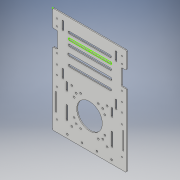
# Autodesk Inventor part: m600frontplate
Saved by Autodesk Inventor 2019 (Build 230136000, 136)
## iProperties
Created: 2019-07-15
Part Number: m600frontplate
Material: Generic
Document SubType Name: Modeling
Designer: Dell
Density: 1 g/cm^3
Appearance: Default
Author: Dell
Autodesk Inventor part; units mm, degrees
ref_plane "YZ Plane" through (0, 0, 0) normal (1, 0, 0) x (0, 1, 0)
ref_plane "XZ Plane" through (0, 0, 0) normal (0, 1, 0) x (-1, 0, 0)
ref_plane "XY Plane" through (0, 0, 0) normal (0, 0, 1) x (1, 0, 0)
sketch "Sketch1" plane through (0, 0, 0) normal (0, 0, 1) x (1, 0, 0)
  line L0 (0, 0) -> (150, 0)
  line L1 (150, 0) -> (150, -215)
  line L2 (150, -215) -> (0, -215)
  line L3 (0, -215) -> (0, 0)
  dimension "d0" = 150
  dimension "d1" = 215
  constraints: 8 end point, 2 parallel, 1 horizontal, 1 perpendicular
  measures "d0" distance of L1.end L2.end
  measures "d1" distance of L0.end L1.end
extrude "Extrusion1" add sketch "Sketch1" along normal blind 2
sketch "Sketch2" plane through (0, 0, 2) normal (0, 0, 1) x (1, 0, 0)
  line L0 (150, 0) -> (0, 0) projected
  line L1 (150, 0) -> (141.16, 0)
  line L2 (141.16, 0) -> (141.16, -27.95)
  line L3 (141.16, -27.95) -> (150, -27.95)
  line L4 (150, -27.95) -> (150, 0)
  line L5 (0, 0) -> (8.84, 0)
  line L6 (8.84, 0) -> (8.84, -27.95)
  line L7 (8.84, -27.95) -> (0, -27.95)
  line L8 (0, -27.95) -> (0, 0)
  line L9 (0, 0) -> (8.84, 0)
  line L10 (8.84, 0) -> (8.84, -13.975)
  line L11 (8.84, -13.975) -> (0, -13.975)
  line L12 (0, -13.975) -> (0, 0)
  line L13 (150, 0) -> (141.16, 0)
  line L14 (141.16, 0) -> (141.16, -13.975)
  line L15 (141.16, -13.975) -> (150, -13.975)
  line L16 (150, -13.975) -> (150, 0)
  circle A0 centre (141.16, -13.975) radius 1.3
  circle A1 centre (141.16, -27.95) radius 1.3
  circle A2 centre (8.84, -13.975) radius 1.3
  circle A3 centre (8.84, -27.95) radius 1.3
  line L17 (0, 0) -> (8.84, 0)
  line L18 (8.84, 0) -> (8.84, -75.2318)
  line L19 (8.84, -75.2318) -> (0, -75.2318)
  line L20 (0, -75.2318) -> (0, 0)
  line L21 (0, 0) -> (0, -215) projected
  line L22 (0, 0) -> (8.84, 0)
  line L23 (8.84, 0) -> (8.84, -95.1591)
  line L24 (8.84, -95.1591) -> (0, -95.1591)
  line L25 (0, -95.1591) -> (0, 0)
  line L26 (0, 0) -> (8.84, 0)
  line L27 (8.84, 0) -> (8.84, -113.5536)
  line L28 (8.84, -113.5536) -> (0, -113.5536)
  line L29 (0, -113.5536) -> (0, 0)
  line L30 (0, 0) -> (8.84, 0)
  line L31 (8.84, 0) -> (8.84, -134.4006)
  line L32 (8.84, -134.4006) -> (0, -134.4006)
  line L33 (0, -134.4006) -> (0, 0)
  line L34 (0, 0) -> (8.84, 0)
  line L35 (8.84, 0) -> (8.84, -192)
  line L36 (8.84, -192) -> (0, -192)
  line L37 (0, -192) -> (0, 0)
  line L38 (150, 0) -> (141.16, 0)
  line L39 (141.16, 0) -> (141.16, -75.2318)
  line L40 (141.16, -75.2318) -> (150, -75.2318)
  line L41 (150, -75.2318) -> (150, 0)
  line L42 (150, 0) -> (141.16, 0)
  line L43 (141.16, 0) -> (141.16, -95.1591)
  line L44 (141.16, -95.1591) -> (150, -95.1591)
  line L45 (150, -95.1591) -> (150, 0)
  line L46 (150, -215) -> (150, 0) projected
  line L47 (150, 0) -> (141.16, 0)
  line L48 (141.16, 0) -> (141.16, -113.5536)
  line L49 (141.16, -113.5536) -> (150, -113.5536)
  line L50 (150, -113.5536) -> (150, 0)
  line L51 (150, 0) -> (141.16, 0)
  line L52 (141.16, 0) -> (141.16, -134.4006)
  line L53 (141.16, -134.4006) -> (150, -134.4006)
  line L54 (150, -134.4006) -> (150, 0)
  line L55 (150, 0) -> (141.16, 0)
  line L56 (141.16, 0) -> (141.16, -192)
  line L57 (141.16, -192) -> (150, -192)
  line L58 (150, -192) -> (150, 0)
  circle A4 centre (8.84, -75.2318) radius 1.3
  circle A5 centre (141.16, -75.2318) radius 1.3
  circle A6 centre (141.16, -95.1591) radius 1.3
  circle A7 centre (8.84, -95.1591) radius 1.3
  circle A8 centre (8.84, -113.5536) radius 1.3
  circle A9 centre (141.16, -113.5536) radius 1.3
  circle A10 centre (141.16, -134.4006) radius 1.3
  circle A11 centre (8.84, -134.4006) radius 1.3
  circle A12 centre (141.16, -192) radius 1.3
  circle A13 centre (8.84, -192) radius 1.3
  line L59 (0, -27.95) -> (10.14, -27.95)
  line L60 (10.14, -27.95) -> (10.14, -34.95)
  line L61 (10.14, -34.95) -> (0, -34.95)
  line L62 (0, -34.95) -> (0, -27.95)
  line L63 (0, -75.2318) -> (10.14, -75.2318)
  line L64 (10.14, -75.2318) -> (10.14, -67.9551)
  line L65 (10.14, -67.9551) -> (0, -67.9551)
  line L66 (0, -67.9551) -> (0, -75.2318)
  line L67 (10.14, -34.95) -> (0, -34.95)
  line L68 (0, -34.95) -> (0, -67.9551)
  line L69 (0, -67.9551) -> (10.14, -67.9551)
  line L70 (10.14, -67.9551) -> (10.14, -34.95)
  line L71 (150, -27.95) -> (139.86, -27.95)
  line L72 (139.86, -27.95) -> (139.86, -34.95)
  line L73 (139.86, -34.95) -> (150, -34.95)
  line L74 (150, -34.95) -> (150, -27.95)
  line L75 (139.86, -34.95) -> (150, -34.95)
  line L76 (150, -34.95) -> (150, -67.9551)
  line L77 (150, -67.9551) -> (139.86, -67.9551)
  line L78 (139.86, -67.9551) -> (139.86, -34.95)
  dimension "d4" = 8.84
  dimension "d5" = 27.95
  dimension "d6" = 8.84
  dimension "d7" = 27.95
  dimension "d8" = 2.6
  dimension "d9" = 2.6
  dimension "d10" = 2.6
  dimension "d11" = 2.6
  dimension "d63" = 192
  dimension "d64" = 2.6
  dimension "d65" = 2.6
  dimension "d66" = 2.6
  dimension "d67" = 2.6
  dimension "d68" = 2.6
  dimension "d69" = 2.6
  dimension "d70" = 2.6
  dimension "d71" = 2.6
  dimension "d72" = 2.6
  dimension "d73" = 2.6
  dimension "d95" = 7
  dimension "d97" = 7
  constraints: 152 end point, 38 parallel, 19 horizontal, 19 perpendicular, 14 centre point, 14 coincident, 8 point on line, 2 midpoint
  measures "d4" distance of L3.end L2.end
  measures "d5" distance of L1.end L2.end
  measures "d6" distance of L6.end L7.end
  measures "d7" distance of L5.end L6.end
  measures "d8" diameter of A0
  measures "d9" diameter of A1
  measures "d10" diameter of A2
  measures "d11" diameter of A3
  measures "d63" distance of L34.end L35.end
  measures "d64" diameter of A4
  measures "d65" diameter of A5
  measures "d66" diameter of A6
  measures "d67" diameter of A7
  measures "d68" diameter of A8
  measures "d69" diameter of A9
  measures "d70" diameter of A10
  measures "d71" diameter of A11
  measures "d72" diameter of A12
  measures "d73" diameter of A13
  measures "d95" distance of L59.end L60.end
  measures "d97" distance of L71.end L72.end
sketch "Sketch3" plane through (0, 0, 2) normal (0, 0, 1) x (1, 0, 0)
  point P0 (0, 0)
sketch "Sketch4" plane through (0, 0, 2) normal (0, 0, 1) x (1, 0, 0)
  line L0 (150, -215) -> (150, 0) projected
  line L1 (150, 0) -> (129.155, 0)
  line L2 (129.155, 0) -> (129.155, -12.875)
  line L3 (129.155, -12.875) -> (150, -12.875)
  line L4 (150, -12.875) -> (150, 0)
  line L5 (0, 0) -> (20.845, 0)
  line L6 (20.845, 0) -> (20.845, -12.875)
  line L7 (20.845, -12.875) -> (0, -12.875)
  line L8 (0, -12.875) -> (0, 0)
  circle A0 centre (129.155, -12.875) radius 1.75
  circle A1 centre (20.845, -12.875) radius 1.75
  line L9 (150, 0) -> (129.155, 0)
  line L10 (129.155, 0) -> (129.155, -97.755)
  line L11 (129.155, -97.755) -> (150, -97.755)
  line L12 (150, -97.755) -> (150, 0)
  line L13 (0, 0) -> (20.845, 0)
  line L14 (20.845, 0) -> (20.845, -97.755)
  line L15 (20.845, -97.755) -> (0, -97.755)
  line L16 (0, -97.755) -> (0, 0)
  circle A2 centre (20.845, -97.755) radius 1.75
  circle A3 centre (129.155, -97.755) radius 1.75
  line L17 (150, 0) -> (0, 0) projected
  line L18 (0, 0) -> (20.845, 0)
  line L19 (20.845, 0) -> (20.845, -27.95)
  line L20 (20.845, -27.95) -> (0, -27.95)
  line L21 (0, -27.95) -> (0, 0)
  circle A4 centre (20.845, -27.95) radius 1.75
  line L22 (150, 0) -> (129.155, 0)
  line L23 (129.155, 0) -> (129.155, -27.95)
  line L24 (129.155, -27.95) -> (150, -27.95)
  line L25 (150, -27.95) -> (150, 0)
  circle A5 centre (129.155, -27.95) radius 1.75
  line L26 (0, -97.755) -> (20.845, -97.755)
  line L27 (20.845, -97.755) -> (20.845, -112.83)
  line L28 (20.845, -112.83) -> (0, -112.83)
  line L29 (0, -112.83) -> (0, -97.755)
  line L30 (150, -97.755) -> (129.155, -97.755)
  line L31 (129.155, -97.755) -> (129.155, -112.83)
  line L32 (129.155, -112.83) -> (150, -112.83)
  line L33 (150, -112.83) -> (150, -97.755)
  circle A6 centre (20.845, -112.83) radius 1.75
  circle A7 centre (129.155, -112.83) radius 1.75
  line L34 (20.845, -12.875) -> (20.845, -27.95) construction
  line L35 (19.095, -12.875) -> (19.095, -27.95)
  line L36 (22.595, -27.95) -> (22.595, -12.875)
  arc A8 (22.595, -12.875) -> (19.095, -12.875) centre (20.845, -12.875) ccw
  arc A9 (19.095, -27.95) -> (22.595, -27.95) centre (20.845, -27.95) ccw
  line L37 (129.155, -27.95) -> (129.1553, -12.8747) construction
  line L38 (130.905, -27.95) -> (130.9053, -12.8747)
  line L39 (127.4053, -12.8746) -> (127.405, -27.95)
  arc A10 (127.405, -27.95) -> (130.905, -27.95) centre (129.155, -27.95) ccw
  arc A11 (130.9053, -12.8747) -> (127.4053, -12.8746) centre (129.1553, -12.8747) ccw
  line L40 (129.155, -97.755) -> (129.155, -112.83) construction
  line L41 (127.405, -97.755) -> (127.405, -112.83)
  line L42 (130.905, -112.83) -> (130.905, -97.755)
  arc A12 (130.905, -97.755) -> (127.405, -97.755) centre (129.155, -97.755) ccw
  arc A13 (127.405, -112.83) -> (130.905, -112.83) centre (129.155, -112.83) ccw
  line L43 (20.845, -97.755) -> (20.845, -112.83) construction
  line L44 (19.095, -97.755) -> (19.095, -112.83)
  line L45 (22.595, -112.83) -> (22.595, -97.755)
  arc A14 (22.595, -97.755) -> (19.095, -97.755) centre (20.845, -97.755) ccw
  arc A15 (19.095, -112.83) -> (22.595, -112.83) centre (20.845, -112.83) ccw
  point P0 (20.845, -20.4125)
  point P1 (129.1551, -20.4123)
  point P2 (129.155, -105.2925)
  point P3 (20.845, -105.2925)
  dimension "d12" = 20.845
  dimension "d13" = 12.875
  dimension "d14" = 20.845
  dimension "d15" = 12.875
  dimension "d16" = 3.5
  dimension "d17" = 3.5
  dimension "d18" = 97.755
  dimension "d19" = 3.5
  dimension "d22" = 3.5
  dimension "d98" = 27.95
  dimension "d99" = 3.5
  dimension "d100" = 27.95
  dimension "d101" = 20.845
  dimension "d102" = 3.5
  dimension "d103" = 97.755
  dimension "d104" = 15.075
  dimension "d105" = 3.5
  dimension "d106" = 3.5
  dimension "d109" = 3.5
  constraints: 96 end point, 20 parallel, 16 centre point, 16 point on circle, 16 tangent, 9 perpendicular, 8 coincident, 8 horizontal, 4 midpoint, 2 collinear, 2 concentric, 1 point on line
  measures "d12" distance of L3.end L2.end
  measures "d13" distance of L1.end L2.end
  measures "d14" distance of L6.end L7.end
  measures "d15" distance of L5.end L6.end
  measures "d16" diameter of A0
  measures "d17" diameter of A1
  measures "d18" distance of L9.end L10.end
  measures "d19" diameter of A2
  measures "d22" diameter of A3
  measures "d98" distance of L18.end L19.end
  measures "d99" diameter of A4
  measures "d100" distance of L22.end L23.end
  measures "d101" distance of L23.end L24.end
  measures "d102" diameter of A5
  measures "d103" distance of L13.end L14.end
  measures "d104" distance of L26.end L27.end
  measures "d105" diameter of A6
  measures "d106" diameter of A7
  measures "d109" diameter of A11
extrude "Extrusion2" cut sketch "Sketch2" against normal blind 2 contours A0 L15 L2 | L2 A0 | A0 L2 L15 | A2 L6 | L6 L11 A2 | A1 L39 L3 | L3 L2 A1 | L41 L77 L39 L73 | L6 A2 L11 | L2 L71 A1 | L39 A1 L71 | L39 L77 L78 L73 | A3 L6 L7 | L7 L18 A3 | L61 L18 L65 L20 | A3 L59 L6 | A5 L43 L40 | L40 L39 A5 | L39 L43 A5 | L59 A3 L18 | L61 L70 L65 L18 | A6 L48 L44 | L44 L43 A6 | L43 L48 A6 | A9 L52 L49 | L49 L48 A9 | A4 L18 L19 | L19 L23 A4 | A4 L63 L18 | L48 L52 A9 | A10 L56 L53 | L53 L52 A10 | L63 A4 L23 | A7 L23 L24 | L24 L27 A7 | A12 L56 L57 | L57 L56 A12 | L56 A10 L52 | A7 L27 L23 | A8 L27 L28 | L28 L31 A8 | A11 L31 L32 | L32 L35 A11 | L27 A8 L31 | A13 L35 L36 | L36 L35 A13 | L31 A11 L35
extrude "Extrusion3" cut sketch "Sketch4" against normal blind 2 contours A7 L31 L32 | L32 L31 A7 | A7 L31 A3 L42 | A3 L31 L11 | L11 L10 A3 | L41 A3 L31 A7 | A5 L10 L24 | L24 L10 A5 | A5 L10 A0 L38 | L31 A3 L10 | A0 L10 L3 | L3 L2 A0 | L10 A5 | A5 L39 A0 L10 | L10 A0 L2 | A1 L14 L6 | L6 L7 A1 | L14 A1 L7 | L36 A4 L14 A1 | A1 L14 A4 L35 | A4 L14 | A4 L14 L20 | L20 L14 A4 | A2 L14 L15 | L15 L27 A2 | A2 L27 A6 L44 | A2 L27 L14 | A2 L45 A6 L27 | A6 L27 L28 | L28 L27 A6
sketch "Sketch5" plane through (0, 0, 2) normal (0, 0, 1) x (1, 0, 0)
  line L0 (33.6074, -26.2636) -> (117.2524, -26.2636) construction
  line L1 (33.6074, -24.0231) -> (117.2524, -24.0231)
  line L2 (117.2524, -28.504) -> (33.6074, -28.504)
  arc A0 (33.6074, -24.0231) -> (33.6074, -28.504) centre (33.6074, -26.2636) ccw
  arc A1 (117.2524, -28.504) -> (117.2524, -24.0231) centre (117.2524, -26.2636) ccw
  point P0 (0, 0)
  point P1 (75.4299, -26.2636)
  constraints: 8 end point, 4 point on circle, 4 tangent, 2 centre point, 1 horizontal, 1 midpoint, 1 parallel
sketch "Sketch6" plane through (0, 0, 2) normal (0, 0, 1) x (1, 0, 0)
  line L0 (34.1053, -37.7772) -> (117.7503, -37.7772) construction
  line L1 (34.1053, -35.5367) -> (117.7503, -35.5367)
  line L2 (117.7503, -40.0177) -> (34.1053, -40.0177)
  arc A0 (34.1053, -35.5367) -> (34.1053, -40.0177) centre (34.1053, -37.7772) ccw
  arc A1 (117.7503, -40.0177) -> (117.7503, -35.5367) centre (117.7503, -37.7772) ccw
  line L3 (34.1053, -37.7772) -> (117.7503, -37.7772) construction
  line L4 (34.1053, -35.5367) -> (117.7503, -35.5367)
  line L5 (117.7503, -40.0177) -> (34.1053, -40.0177)
  arc A2 (34.1053, -35.5367) -> (34.1053, -40.0177) centre (34.1053, -37.7772) ccw
  arc A3 (117.7503, -40.0177) -> (117.7503, -35.5367) centre (117.7503, -37.7772) ccw
  point P0 (0, 0)
  point P1 (75.9278, -37.7772)
  point P2 (0, 0)
  point P3 (75.9278, -37.7772)
  constraints: 16 end point, 8 point on circle, 8 tangent, 4 centre point, 2 horizontal, 2 midpoint, 2 parallel
sketch "Sketch7" plane through (0, 0, 2) normal (0, 0, 1) x (1, 0, 0)
  line L0 (34.1053, -37.7772) -> (117.7503, -37.7772) construction
  line L1 (34.1053, -35.5367) -> (117.7503, -35.5367)
  line L2 (117.7503, -40.0177) -> (34.1053, -40.0177)
  arc A0 (34.1053, -35.5367) -> (34.1053, -40.0177) centre (34.1053, -37.7772) ccw
  arc A1 (117.7503, -40.0177) -> (117.7503, -35.5367) centre (117.7503, -37.7772) ccw
  line L3 (34.1053, -37.7772) -> (117.7503, -37.7772) construction
  line L4 (34.1053, -35.5367) -> (117.7503, -35.5367)
  line L5 (117.7503, -40.0177) -> (34.1053, -40.0177)
  arc A2 (34.1053, -35.5367) -> (34.1053, -40.0177) centre (34.1053, -37.7772) ccw
  arc A3 (117.7503, -40.0177) -> (117.7503, -35.5367) centre (117.7503, -37.7772) ccw
  point P0 (0, 0)
  point P1 (75.9278, -37.7772)
  point P2 (0, 0)
  point P3 (75.9278, -37.7772)
  constraints: 16 end point, 8 point on circle, 8 tangent, 4 centre point, 2 horizontal, 2 midpoint, 2 parallel
sketch "Sketch8" plane through (0, 0, 2) normal (0, 0, 1) x (1, 0, 0)
  line L0 (34.1053, -74.2842) -> (117.7503, -74.2842) construction
  line L1 (34.1053, -72.0437) -> (117.7503, -72.0437)
  line L2 (117.7503, -76.5246) -> (34.1053, -76.5246)
  arc A0 (34.1053, -72.0437) -> (34.1053, -76.5246) centre (34.1053, -74.2842) ccw
  arc A1 (117.7503, -76.5246) -> (117.7503, -72.0437) centre (117.7503, -74.2842) ccw
  line L3 (34.1053, -84.5028) -> (117.7503, -84.5028) construction
  line L4 (34.1053, -82.2623) -> (117.7503, -82.2623)
  line L5 (117.7503, -86.7433) -> (34.1053, -86.7433)
  arc A2 (34.1053, -82.2623) -> (34.1053, -86.7433) centre (34.1053, -84.5028) ccw
  arc A3 (117.7503, -86.7433) -> (117.7503, -82.2623) centre (117.7503, -84.5028) ccw
  point P0 (0, 0)
  point P1 (75.9278, -74.2842)
  point P2 (0, 0)
  point P3 (75.9278, -84.5028)
  constraints: 16 end point, 8 point on circle, 8 tangent, 4 centre point, 2 horizontal, 2 midpoint, 2 parallel
sketch "Sketch9" plane through (0, 0, 2) normal (0, 0, 1) x (1, 0, 0)
  line L0 (34.1053, -48.7434) -> (117.7503, -48.7434) construction
  line L1 (34.1053, -46.5029) -> (117.7503, -46.5029)
  line L2 (117.7503, -50.9839) -> (34.1053, -50.9839)
  arc A0 (34.1053, -46.5029) -> (34.1053, -50.9839) centre (34.1053, -48.7434) ccw
  arc A1 (117.7503, -50.9839) -> (117.7503, -46.5029) centre (117.7503, -48.7434) ccw
  line L3 (34.1053, -61.1223) -> (117.7503, -61.1223) construction
  line L4 (34.1053, -58.8818) -> (117.7503, -58.8818)
  line L5 (117.7503, -63.3628) -> (34.1053, -63.3628)
  arc A2 (34.1053, -58.8818) -> (34.1053, -63.3628) centre (34.1053, -61.1223) ccw
  arc A3 (117.7503, -63.3628) -> (117.7503, -58.8818) centre (117.7503, -61.1223) ccw
  point P0 (0, 0)
  point P1 (75.9278, -48.7434)
  point P2 (0, 0)
  point P3 (75.9278, -61.1223)
  constraints: 16 end point, 8 point on circle, 8 tangent, 4 centre point, 2 horizontal, 2 midpoint, 2 parallel
extrude "Extrusion4" cut sketch "Sketch5" against normal blind 2
extrude "Extrusion5" cut sketch "Sketch8" against normal blind 2 contours L4 A3 L5 A2
extrude "Extrusion6" cut sketch "Sketch9" against normal blind 2 contours L1 A1 L2 A0
extrude "Extrusion7" cut sketch "Sketch7" against normal blind 2
sketch "Sketch10" plane through (0, 0, 2) normal (0, 0, 1) x (1, 0, 0)
  point P0 (0, 0)
sketch "Sketch11" plane through (0, 0, 2) normal (0, 0, 1) x (1, 0, 0)
  line L0 (33.6132, -65.4654) -> (118.088, -65.4654) construction
  line L1 (33.6132, -62.7798) -> (118.088, -62.7798)
  line L2 (118.088, -68.151) -> (33.6132, -68.151)
  arc A0 (33.6132, -62.7798) -> (33.6132, -68.151) centre (33.6132, -65.4654) ccw
  arc A1 (118.088, -68.151) -> (118.088, -62.7798) centre (118.088, -65.4654) ccw
  point P0 (0, 0)
  point P1 (75.8506, -65.4654)
  constraints: 8 end point, 4 point on circle, 4 tangent, 2 centre point, 1 horizontal, 1 midpoint, 1 parallel
extrude "Extrusion8" cut sketch "Sketch11" against normal blind 2
sketch "Sketch12" plane through (0, 0, 2) normal (0, 0, 1) x (1, 0, 0)
  line L0 (0, 0) -> (150, 0) projected
  line L1 (75, 0) -> (75, -153.1)
  line L2 (57, -184.28) -> (93, -184.28)
  line L3 (93, -184.28) -> (93, -121.92)
  line L4 (93, -121.92) -> (57, -121.92)
  line L5 (57, -121.92) -> (57, -184.28)
  line L6 (57, -184.28) -> (93, -121.92) construction
  line L7 (93, -184.28) -> (57, -121.92) construction
  circle A0 centre (93, -121.92) radius 1.75
  circle A1 centre (57, -121.92) radius 1.75
  circle A2 centre (93, -184.28) radius 1.75
  circle A3 centre (57, -184.28) radius 1.75
  line L8 (43.82, -171.1) -> (106.18, -171.1)
  line L9 (106.18, -171.1) -> (106.18, -135.1)
  line L10 (106.18, -135.1) -> (43.82, -135.1)
  line L11 (43.82, -135.1) -> (43.82, -171.1)
  line L12 (43.82, -171.1) -> (106.18, -135.1) construction
  line L13 (106.18, -171.1) -> (43.82, -135.1) construction
  circle A4 centre (106.18, -135.1) radius 1.75
  circle A5 centre (43.82, -135.1) radius 1.75
  circle A6 centre (106.18, -171.1) radius 1.75
  circle A7 centre (43.82, -171.1) radius 1.75
  line L14 (48, -180.1) -> (102, -180.1)
  line L15 (102, -180.1) -> (102, -126.1)
  line L16 (102, -126.1) -> (48, -126.1)
  line L17 (48, -126.1) -> (48, -180.1)
  line L18 (48, -180.1) -> (102, -126.1) construction
  line L19 (102, -180.1) -> (48, -126.1) construction
  circle A8 centre (102, -126.1) radius 1.8
  circle A9 centre (48, -126.1) radius 1.75
  circle A10 centre (102, -180.1) radius 1.75
  circle A11 centre (48, -180.1) radius 1.75
  line L20 (39, -189.1) -> (111, -189.1)
  line L21 (111, -189.1) -> (111, -117.1)
  line L22 (111, -117.1) -> (39, -117.1)
  line L23 (39, -117.1) -> (39, -189.1)
  line L24 (39, -189.1) -> (111, -117.1) construction
  line L25 (111, -189.1) -> (39, -117.1) construction
  circle A12 centre (111, -117.1) radius 1.75
  circle A13 centre (39, -117.1) radius 1.75
  circle A14 centre (111, -189.1) radius 1.75
  circle A15 centre (39, -189.1) radius 1.75
  circle A16 centre (75, -153.1) radius 26
  line L26 (32.5, -195.6) -> (117.5, -195.6)
  line L27 (117.5, -195.6) -> (117.5, -110.6)
  line L28 (117.5, -110.6) -> (32.5, -110.6)
  line L29 (32.5, -110.6) -> (32.5, -195.6)
  line L30 (32.5, -195.6) -> (117.5, -110.6) construction
  line L31 (117.5, -195.6) -> (32.5, -110.6) construction
  line L32 (6.7861, -144.5289) -> (6.7861, -179.5289) construction
  line L33 (5.7861, -144.5289) -> (5.7861, -179.5289)
  line L34 (7.7861, -179.5289) -> (7.7861, -144.5289)
  arc A17 (7.7861, -144.5289) -> (5.7861, -144.5289) centre (6.7861, -144.5289) ccw
  arc A18 (5.7861, -179.5289) -> (7.7861, -179.5289) centre (6.7861, -179.5289) ccw
  line L35 (29.0837, -157.4682) -> (29.0837, -182.4682) construction
  line L36 (27.4337, -157.4682) -> (27.4337, -182.4682)
  line L37 (30.7337, -182.4682) -> (30.7337, -157.4682)
  arc A19 (30.7337, -157.4682) -> (27.4337, -157.4682) centre (29.0837, -157.4682) ccw
  arc A20 (27.4337, -182.4682) -> (30.7337, -182.4682) centre (29.0837, -182.4682) ccw
  line L38 (143.5364, -179.5289) -> (143.5364, -144.5289) construction
  line L39 (144.5364, -179.5289) -> (144.5364, -144.5289)
  line L40 (142.5364, -144.5289) -> (142.5364, -179.5289)
  arc A21 (142.5364, -179.5289) -> (144.5364, -179.5289) centre (143.5364, -179.5289) ccw
  arc A22 (144.5364, -144.5289) -> (142.5364, -144.5289) centre (143.5364, -144.5289) ccw
  line L41 (120.8663, -183.6569) -> (120.8663, -158.6569) construction
  line L42 (150, 0) -> (150, -215) projected
  line L43 (122.5163, -183.6569) -> (122.5163, -158.6569)
  line L44 (119.2163, -158.6569) -> (119.2163, -183.6569)
  arc A23 (119.2163, -183.6569) -> (122.5163, -183.6569) centre (120.8663, -183.6569) ccw
  arc A24 (122.5163, -158.6569) -> (119.2163, -158.6569) centre (120.8663, -158.6569) ccw
  line L45 (28.9774, -116.6542) -> (28.9774, -130.6542) construction
  line L46 (27.3774, -116.6542) -> (27.3774, -130.6542)
  line L47 (30.5774, -130.6542) -> (30.5774, -116.6542)
  arc A25 (30.5774, -116.6542) -> (27.3774, -116.6542) centre (28.9774, -116.6542) ccw
  arc A26 (27.3774, -130.6542) -> (30.5774, -130.6542) centre (28.9774, -130.6542) ccw
  line L48 (120.8663, -116.6231) -> (120.8663, -130.6231) construction
  line L49 (119.2163, -116.6231) -> (119.2163, -130.6231)
  line L50 (122.5163, -130.6231) -> (122.5163, -116.6231)
  arc A27 (122.5163, -116.6231) -> (119.2163, -116.6231) centre (120.8663, -116.6231) ccw
  arc A28 (119.2163, -130.6231) -> (122.5163, -130.6231) centre (120.8663, -130.6231) ccw
  point P0 (6.7861, -162.0289)
  point P1 (29.0837, -169.9682)
  point P2 (143.5364, -162.0289)
  point P3 (120.8663, -171.1569)
  point P4 (28.9774, -123.6542)
  point P5 (120.8663, -123.6231)
  dimension "d35" = 153.1
  dimension "d36" = 36
  dimension "d37" = 62.36
  dimension "d38" = 3.5
  dimension "d39" = 3.5
  dimension "d40" = 3.5
  dimension "d41" = 3.5
  dimension "d42" = 62.36
  dimension "d43" = 36
  dimension "d44" = 3.5
  dimension "d45" = 3.5
  dimension "d46" = 3.5
  dimension "d47" = 3.5
  dimension "d48" = 54
  dimension "d49" = 54
  dimension "d50" = 3.6
  dimension "d51" = 3.5
  dimension "d52" = 3.5
  dimension "d53" = 3.5
  dimension "d54" = 72
  dimension "d55" = 72
  dimension "d56" = 3.5
  dimension "d57" = 3.5
  dimension "d58" = 3.5
  dimension "d59" = 3.5
  dimension "d60" = 52
  dimension "d85" = 85
  dimension "d86" = 85
  dimension "d87" = 2
  dimension "d88" = 3.3
  dimension "d89" = 2
  dimension "d90" = 3.3
  dimension "d91" = 25
  dimension "d92" = 25
  dimension "d93" = 3.2
  dimension "d94" = 3.3
  dimension "d107" = 14
  dimension "d108" = 14
  dimension "d110" = 35
  dimension "d111" = 35
  constraints: 110 end point, 29 centre point, 24 point on circle, 24 tangent, 20 parallel, 17 coincident, 17 midpoint, 5 horizontal, 5 perpendicular, 3 vertical
  measures "d35" distance of L1.start L1.end
  measures "d36" distance of L4.end L3.end
  measures "d37" distance of L2.end L3.end
  measures "d38" diameter of A0
  measures "d39" diameter of A1
  measures "d40" diameter of A2
  measures "d41" diameter of A3
  measures "d42" distance of L10.end L9.end
  measures "d43" distance of L8.end L9.end
  measures "d44" diameter of A4
  measures "d45" diameter of A5
  measures "d46" diameter of A6
  measures "d47" diameter of A7
  measures "d48" distance of L16.end L15.end
  measures "d49" distance of L14.end L15.end
  measures "d50" diameter of A8
  measures "d51" diameter of A9
  measures "d52" diameter of A10
  measures "d53" diameter of A11
  measures "d54" distance of L22.end L21.end
  measures "d55" distance of L20.end L21.end
  measures "d56" diameter of A12
  measures "d57" diameter of A13
  measures "d58" diameter of A14
  measures "d59" diameter of A15
  measures "d60" diameter of A16
  measures "d85" distance of L28.end L27.end
  measures "d86" distance of L28.end L26.start
  measures "d87" diameter of A18
  measures "d88" diameter of A20
  measures "d89" diameter of A22
  measures "d90" diameter of A24
  measures "d91" distance of L35.start L35.end
  measures "d92" distance of L41.start L41.end
  measures "d93" diameter of A26
  measures "d94" diameter of A28
  measures "d107" distance of L46.start L46.end
  measures "d108" distance of L50.start L50.end
  measures "d110" distance of L34.start L34.end
  measures "d111" distance of L39.start L39.end
extrude "Extrusion9" cut sketch "Sketch12" against normal blind 2 contours A12 L21 L22 | L22 L21 A12 | A13 L23 L22 | L22 L23 A13 | A0 L3 L4 | L4 L3 A0 | A1 L5 L4 | L4 L5 A1 | A16 L3 L10 L1 | L1 L10 L5 A16 | A14 L20 L21 | L21 L20 A14 | A15 L20 L23 | L23 L20 A15 | L10 L3 L8 L5 | A16 L10 L3 | L5 L10 A16 | A8 L15 L16 | L16 L15 A8 | A9 L17 L16 | L16 L17 A9 | L10 A16 L8 L3 | L5 L8 A16 L10 | L8 A16 L3 | L3 A16 L5 L8 | L5 A16 L8 | A4 L9 L10 | L10 L9 A4 | A5 L11 L10 | L10 L11 A5 | A6 L9 L8 | L8 L9 A6 | A10 L14 L15 | L15 L14 A10 | A7 L11 L8 | L8 L11 A7 | A11 L14 L17 | L17 L14 A11 | A2 L2 L3 | L3 L2 A2 | A3 L2 L5 | L5 L2 A3 | A17 L34 A18 L33 | A19 L37 A20 L36 | A21 L40 A22 L39 | A23 L44 A24 L43 | A25 L47 A26 L46 | A27 L50 A28 L49
sketch "Sketch13" plane through (0, 0, 2) normal (0, 0, 1) x (1, 0, 0)
  line L0 (0, -215) -> (150, -215) projected
  line L1 (0, -215) -> (30, -215)
  line L2 (30, -215) -> (30, -207.5)
  line L3 (30, -207.5) -> (0, -207.5)
  line L4 (0, -207.5) -> (0, -215)
  line L5 (30, -207.5) -> (60, -207.5)
  line L6 (60, -207.5) -> (60, -215)
  line L7 (60, -215) -> (30, -215)
  line L8 (30, -215) -> (30, -207.5)
  line L9 (60, -207.5) -> (90, -207.5)
  line L10 (90, -207.5) -> (90, -215)
  line L11 (90, -215) -> (60, -215)
  line L12 (60, -215) -> (60, -207.5)
  line L13 (90, -207.5) -> (120, -207.5)
  line L14 (120, -207.5) -> (120, -215)
  line L15 (120, -215) -> (90, -215)
  line L16 (90, -215) -> (90, -207.5)
  circle A0 centre (30, -207.5) radius 1.75
  circle A1 centre (60, -207.5) radius 1.75
  circle A2 centre (90, -207.5) radius 1.75
  circle A3 centre (120, -207.5) radius 1.75
  point P0 (0, 0)
  dimension "d74" = 7.5
  dimension "d75" = 30
  dimension "d76" = 30
  dimension "d77" = 30
  dimension "d78" = 30
  dimension "d79" = 3.5
  dimension "d80" = 3.5
  dimension "d81" = 3.5
  dimension "d82" = 3.5
  constraints: 32 end point, 8 parallel, 4 centre point, 4 coincident, 4 horizontal, 4 perpendicular, 3 point on line
  measures "d74" distance of L1.end L2.end
  measures "d75" distance of L2.end L3.end
  measures "d76" distance of L6.end L7.end
  measures "d77" distance of L10.end L11.end
  measures "d78" distance of L14.end L15.end
  measures "d79" diameter of A0
  measures "d80" diameter of A1
  measures "d81" diameter of A2
  measures "d82" diameter of A3
extrude "Extrusion10" cut sketch "Sketch13" against normal blind 2 contours A0 L3 L2 | L2 L5 A0 | A0 L5 L3 | A1 L5 L6 | L6 L9 A1 | A2 L9 L10 | L10 L13 A2 | L5 A1 L9 | A3 L13 L14 | L14 L13 A3 | L9 A2 L13
fillet "Fillet1" radius 2 12 edges at (139.86, -34.95, 1) (150, -34.95, 1) (150, -67.9551, 1) (139.86, -67.9551, 1) (10.14, -67.9551, 1) (0, -67.9551, 1) (0, -34.95, 1) (10.14, -34.95, 1) (150, 0, 1) (0, 0, 1) (150, -215, 1) (0, -215, 1)
body "Solid1"
